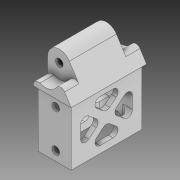
# Autodesk Inventor part: 254 Billet Top Block
Saved by Autodesk Inventor 2021 (Build 250183000, 183)
## iProperties
Created: 2021-03-21
Part Number: 254 Billet Top Block
Material: Generic
Document SubType Name: Modeling
Density: 1 g/cm^3
Appearance: Default
Autodesk Inventor part; units mm, degrees
ref_plane "YZ Plane" through (0, 0, 0) normal (1, 0, 0) x (0, 1, 0)
ref_plane "XZ Plane" through (0, 0, 0) normal (0, 1, 0) x (-1, 0, 0)
ref_plane "XY Plane" through (0, 0, 0) normal (0, 0, 1) x (1, 0, 0)
sketch "Sketch1" plane through (0, 0, 0) normal (0, 0, 1) x (1, 0, 0)
  line L0 (-13.4938, 19.05) -> (-11.9063, 19.05)
  line L1 (-11.9063, 19.05) -> (-11.9063, -19.05)
  line L2 (-11.9063, -19.05) -> (10.3187, -19.05)
  line L3 (10.3187, -19.05) -> (10.3187, 19.05)
  line L4 (10.3187, 19.05) -> (11.9062, 19.05)
  line L5 (11.9062, 19.05) -> (1.1453, 36.0037)
  arc A0 (1.1453, 36.0037) -> (-13.4938, 31.75) centre (-5.5563, 31.75) ccw
  line L6 (-13.4938, 31.75) -> (-13.4938, 19.05)
  circle A1 centre (-5.5563, 31.75) radius 2.5527
  circle A2 centre (-5.5563, 31.75) radius 9.525 construction
  line L7 (-15.0813, 37.5649) -> (-15.0813, -31.0357) construction
  line L8 (-11.9063, -19.05) -> (11.9062, 19.05) construction
  circle A3 centre (0, 12.7) radius 2.5527
  line L9 (0, 0) -> (19.8072, 0)
  circle A4 centre (0, -12.7) radius 2.5527
  dimension "d0" = 25.4
  dimension "d1" = 1.5875
  dimension "d2" = 38.1
  dimension "d3" = 5.1054
  dimension "d4" = 19.05
  dimension "d5" = 1.5875
  dimension "d6" = 12.7
  dimension "d7" = 15.875
  dimension "d8" = 5.1054
  dimension "d10" = 25.4
  constraints: 20 end point, 5 centre point, 4 perpendicular, 3 coincident, 3 tangent, 2 collinear, 2 horizontal, 2 point on circle, 1 midpoint, 1 symmetric about line, 1 vertical, 1 vertical alignment, 1 other
  measures "d0" distance of L4.end L0.start
  measures "d1" distance from line of L4.end L3
  measures "d2" distance from line of L3.end L2
  measures "d3" diameter of A1
  measures "d4" diameter of A2
  measures "d5" distance from line of L0.start L7
  measures "d6" distance from line of L0 A0.centre
  measures "d7" diameter of A0
  measures "d8" diameter of A3
  measures "d10" distance of A4.centre A3.centre
extrude "Extrusion1" add sketch "Sketch1" along normal mid plane 50.8
sketch "Sketch2" plane through (-11.9063, -19.05, 25.4) normal (0, -1, 0) x (1, 0, 0)
  line L0 (0, 0) -> (22.225, 0) projected
  line L1 (22.225, -50.8) -> (0, -50.8) projected
  line L2 (0, -1.5875) -> (22.225, -1.5875)
  line L3 (22.225, -49.2125) -> (0, -49.2125)
  line L4 (22.225, 0) -> (22.225, -50.8) projected
  line L5 (0, 0) -> (22.225, 0) projected
  line L6 (0, -50.8) -> (0, 0) projected
  line L7 (22.225, -50.8) -> (0, -50.8) projected
  point P0 (11.9063, -25.4)
  point P1 (0, -1.5875)
  point P2 (22.225, -1.5875)
  dimension "d13" = 1.5875
  dimension "d14" = 1.5875
  constraints: 4 end point, 2 parallel
  measures "d13" distance between parallel lines of L1 L3
  measures "d14" distance between parallel lines of L0 L2
extrude "Extrusion2" cut sketch "Sketch2" against normal up to surface (38.1 mm away) contours L0 L4 L2 L6 | L3 L4 L1 L6
sketch "Sketch3" plane through (0, 0, -25.4) normal (0, 0, -1) x (-1, 0, 0)
  circle A0 centre (5.5563, 31.75) radius 2.5527 projected
  line L0 (-11.9062, 19.05) -> (13.4938, 19.05) projected
  line L1 (13.4938, 19.05) -> (13.4938, 31.75) projected
  arc A1 (13.4938, 31.75) -> (-1.1453, 36.0037) centre (5.5563, 31.75) ccw projected
  line L2 (-1.1453, 36.0037) -> (-11.9062, 19.05) projected
  circle A2 centre (5.5563, 31.75) radius 9.6044
  point P0 (0, 0)
  point P1 (-4.0431, 31.4382)
  point P2 (13.4938, 26.3426)
  dimension "d17" = 19.2087
  constraints: 1 centre point, 1 coincident
  measures "d17" diameter of A2
extrude "Extrusion3" cut sketch "Sketch3" against normal blind 9.525 contours L2 A1 L1 A2 picked at (-0.7282, 33.064)
mirror "Mirror1" about plane through (0, 0, 0) normal (0, 0, 1) of "Extrusion3"
fillet "Fillet1" radius 3.175 4 edges at (4.0431, 31.4382, -20.6375) (-13.4938, 26.3426, -20.6375) (4.0431, 31.4382, 20.6375) (-13.4938, 26.3426, 20.6375)
sketch "Sketch4" plane through (-11.9063, -19.05, -23.8125) normal (0, -1, 0) x (1, 0, 0)
  line L0 (0, 0) -> (22.225, 0) projected
  line L1 (22.225, 47.625) -> (22.225, 0) projected
  line L2 (22.225, 47.625) -> (0, 47.625) projected
  line L3 (0, 0) -> (0, 47.625) projected
  line L4 (19.05, 41.275) -> (3.175, 41.275)
  line L5 (3.175, 41.275) -> (3.175, 6.35)
  line L6 (3.175, 6.35) -> (19.05, 6.35)
  line L7 (19.05, 6.35) -> (19.05, 41.275)
  dimension "d22" = 3.175
  dimension "d23" = 3.175
  dimension "d24" = 6.35
  dimension "d25" = 6.35
  constraints: 8 end point, 2 parallel, 1 horizontal, 1 perpendicular
  measures "d22" distance between parallel lines of L1 L7
  measures "d23" distance between parallel lines of L3 L5
  measures "d24" distance between parallel lines of L0 L6
  measures "d25" distance between parallel lines of L2 L4
extrude "Extrusion4" cut sketch "Sketch4" against normal up to surface (38.1 mm away) contours L7 L6 L5 L4
sketch "Sketch5" plane through (10.3187, -19.05, -23.8125) normal (1, 0, 0) x (0, 0, -1)
  line L0 (0, 0) -> (0, 38.1) projected
  line L1 (0, 38.1) -> (-47.625, 38.1) projected
  line L2 (-47.625, 38.1) -> (-47.625, 0) projected
  line L3 (-47.625, 0) -> (0, 0) projected
  line L4 (-6.35, 38.1) -> (-41.275, 38.1) projected
  line L5 (-41.275, 0) -> (-41.275, 38.1) projected
  line L6 (-6.35, 0) -> (-41.275, 0) projected
  line L7 (-6.35, 0) -> (-6.35, 38.1) projected
  line L8 (-47.625, 38.1) -> (-47.625, 0) projected
  line L9 (-47.625, 33.3375) -> (0, 33.3375)
  line L10 (0, 38.1) -> (0, 0) projected
  line L11 (-47.625, 4.7625) -> (0, 4.7625)
  line L12 (-6.35, 0) -> (-6.35, 38.1) projected
  line L13 (-6.35, 33.3375) -> (-41.275, 4.7625) construction
  line L14 (-41.275, 3.7973) -> (-41.275, 8.9027) projected
  line L15 (-7.8579, 35.1805) -> (-42.7829, 6.6055)
  line L16 (-39.7671, 2.9195) -> (-4.8421, 31.4945)
  arc A0 (-4.8421, 31.4945) -> (-7.8579, 35.1805) centre (-6.35, 33.3375) ccw
  arc A1 (-42.7829, 6.6055) -> (-39.7671, 2.9195) centre (-41.275, 4.7625) ccw
  line L17 (-41.275, 33.3375) -> (-6.35, 4.7625) construction
  line L18 (-42.7829, 31.4945) -> (-7.8579, 2.9195)
  line L19 (-4.8421, 6.6055) -> (-39.7671, 35.1805)
  arc A2 (-39.7671, 35.1805) -> (-42.7829, 31.4945) centre (-41.275, 33.3375) ccw
  arc A3 (-7.8579, 2.9195) -> (-4.8421, 6.6055) centre (-6.35, 4.7625) ccw
  point P0 (-23.8125, 19.05)
  point P1 (-23.8125, 19.05)
  point P2 (-23.8125, 19.05)
  point P3 (-37.5146, 33.3375)
  point P4 (-23.8125, 22.1267)
  point P5 (-10.1104, 33.3375)
  point P6 (-20.0521, 19.05)
  point P7 (-6.35, 7.8392)
  point P8 (-6.35, 30.2608)
  point P9 (-10.1104, 4.7625)
  point P10 (-23.8125, 15.9733)
  point P11 (-37.5146, 4.7625)
  point P12 (-27.5729, 19.05)
  point P13 (-41.275, 30.2608)
  point P14 (-41.275, 7.8392)
  dimension "d29" = 4.7625
  dimension "d30" = 4.7625
  dimension "d31" = 4.7625
  dimension "d32" = 4.7625
  constraints: 20 end point, 12 point on line, 8 point on circle, 8 tangent, 4 centre point, 2 midpoint, 2 parallel, 2 perpendicular
  measures "d29" distance between parallel lines of L3 L11
  measures "d30" distance between parallel lines of L1 L9
  measures "d31" diameter of A1
  measures "d32" diameter of A3
extrude "Extrusion5" cut sketch "Sketch5" against normal through all contours L19 L16 L7 | L11 L16 L18 | L15 L19 L9 | L15 L5 L18
fillet "Fillet3" radius 3.302 24 edges at (8.7312, 0, -3.7604) (-10.3188, 0, -3.7604) (8.7313, -14.2875, -13.7021) (8.7312, -3.0767, 0) (-10.3188, -3.0767, 0) (-10.3188, -14.2875, -13.7021) (8.7312, -14.2875, 13.7021) (-10.3188, -14.2875, 13.7021) (8.7312, 14.2875, 13.7021) (8.7312, 3.0767, 0) (-10.3188, 3.0767, 0) (-10.3188, 14.2875, 13.7021) (8.7313, 14.2875, -13.7021) (-10.3188, 14.2875, -13.7021) (8.7312, 0, 3.7604) (-10.3188, 0, 3.7604) (8.7313, -11.2108, -17.4625) (8.7312, -11.2108, 17.4625) (-10.3188, -11.2108, 17.4625) (-10.3188, -11.2108, -17.4625) (8.7312, 11.2108, 17.4625) (8.7313, 11.2108, -17.4625) (-10.3188, 11.2108, -17.4625) (-10.3188, 11.2108, 17.4625)
fillet "Fillet2" radius 3.302 12 edges at (7.1437, 7.7268, 17.4625) (7.1437, -15.1304, 17.4625) (7.1437, -7.7268, 17.4625) (-8.7312, -15.1304, -17.4625) (-8.7312, 7.7268, -17.4625) (-8.7312, -7.7268, -17.4625) (7.1438, -7.7268, -17.4625) (7.1438, -15.1304, -17.4625) (7.1438, 7.7268, -17.4625) (-8.7313, -15.1304, 17.4625) (-8.7313, -7.7268, 17.4625) (-8.7313, 7.7268, 17.4625)
equation "\"d14\" = d13"
equation "\"d23\" = d22"
equation "\"d25\" = d24"
equation "\"d30\" = d29"
body "Solid1"
